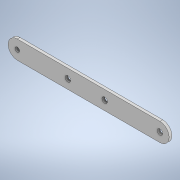
# Autodesk Inventor part: glowny_wahacz
Saved by Autodesk Inventor 2020.3 (Build 243373000, 373)
## iProperties
Created: 2021-10-24
Part Number: glowny_wahacz
Material: Ogólny
Document SubType Name: Modeling
Designer: patry
Density: 1 g/cm^3
Appearance: Domyślna
Author: patry
Autodesk Inventor part; units mm, degrees
ref_plane "YZ Plane" through (0, 0, 0) normal (1, 0, 0) x (0, 1, 0)
ref_plane "XZ Plane" through (0, 0, 0) normal (0, 1, 0) x (-1, 0, 0)
ref_plane "XY Plane" through (0, 0, 0) normal (0, 0, 1) x (1, 0, 0)
sketch "Szkic1" plane through (0, 0, 0) normal (0, 0, 1) x (1, 0, 0)
  line L0 (0, 0) -> (155, 0) construction
  line L1 (0, -10) -> (155, -10)
  line L2 (155, 10) -> (0, 10)
  arc A0 (0, 10) -> (0, -10) centre (0, 0) ccw
  arc A1 (155, -10) -> (155, 10) centre (155, 0) ccw
  point P0 (77.5, 0)
  point P1 (95, 0)
  point P2 (55, 0)
  dimension "d0" = 155
  dimension "d1" = 20
  dimension "d2" = 60
  dimension "d12" = 55
  constraints: 8 end point, 4 point on circle, 4 tangent, 2 centre point, 2 coincident, 2 point on line, 1 horizontal, 1 midpoint, 1 parallel
  measures "d0" distance of L0.start L0.end
  measures "d1" diameter of A1
  measures "d2" distance of point (155, 0) point (95, 0)
  measures "d12" distance of point (0, 0) point (55, 0)
extrude "Wyciągnięcie proste1" add sketch "Szkic1" along normal blind 3
hole "Otwór1" at (155, 0, 0) at (95, 0, 0) at (55, 0, 0) direction (0, 0, 1) diameter 6 end through all
hole "Otwór2" at (0, 0, 0) direction (0, 0, 1) diameter 5 end through all
